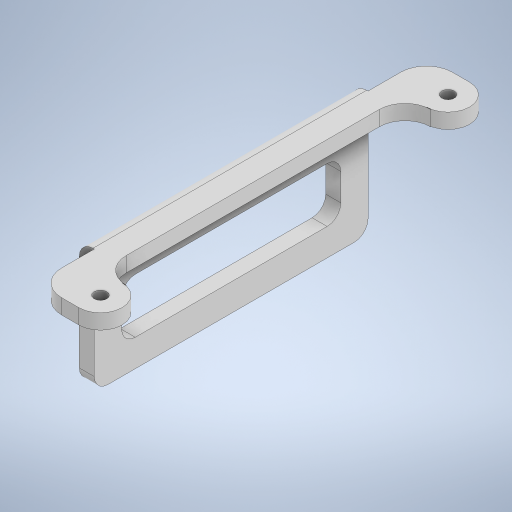
# Autodesk Inventor part: sidemount3
Saved by Autodesk Inventor 2023 (Build 270158000, 158)
## iProperties
Created: 2022-12-04
Part Number: sidemount3
Material: Generic
Document SubType Name: Modeling
Designer: user
Density: 1 g/cm^3
Appearance: Default
Author: user
Autodesk Inventor part; units mm, degrees
ref_plane "YZ Plane" through (0, 0, 0) normal (1, 0, 0) x (0, 1, 0)
ref_plane "XZ Plane" through (0, 0, 0) normal (0, 1, 0) x (-1, 0, 0)
ref_plane "XY Plane" through (0, 0, 0) normal (0, 0, 1) x (1, 0, 0)
sketch "Sketch1" plane through (0, 0, 0) normal (0, 1, 0) x (-1, 0, 0)
  circle A0 centre (0, 0) radius 1.4732
  circle A1 centre (0, -80.9498) radius 1.4732
  circle A2 centre (0, 0) radius 5.0165
  circle A3 centre (0, -80.9498) radius 5.0165
  line L0 (0, 5.0165) -> (4.033, 5.0165)
  line L1 (4.033, -85.9663) -> (0, -85.9663)
  line L2 (10.033, -79.9663) -> (10.033, -0.9835)
  line L3 (0, -5.0165) -> (-0.9835, -5.0165)
  line L4 (5.0165, -11.0165) -> (5.0165, -69.9333)
  line L5 (-0.9835, -75.9333) -> (0, -75.9333)
  arc A4 (10.033, -0.9835) -> (4.033, 5.0165) centre (4.033, -0.9835) ccw
  arc A5 (4.033, -85.9663) -> (10.033, -79.9663) centre (4.033, -79.9663) ccw
  arc A6 (5.0165, -11.0165) -> (-0.9835, -5.0165) centre (-0.9835, -11.0165) ccw
  arc A7 (-0.9835, -75.9333) -> (5.0165, -69.9333) centre (-0.9835, -69.9333) ccw
  point P0 (10.033, 5.0165)
  dimension "d0" = 2.9464
  dimension "d2" = 2.9464
  dimension "d3" = 10.033
  dimension "d4" = 10.033
  dimension "d7" = 80.9498
  dimension "d8" = 10.033
  dimension "d9" = 6
  dimension "d10" = 6
  dimension "d11" = 6
  dimension "d12" = 6
  constraints: 12 end point, 12 point on circle, 11 tangent, 8 centre point, 3 coincident, 2 perpendicular, 2 point on line, 1 horizontal
  measures "d0" diameter of A0
  measures "d2" diameter of A1
  measures "d3" diameter of A2
  measures "d4" diameter of A3
  measures "d7" distance of A2.centre A3.centre
  measures "d8" distance of L0.start point (10.033, 5.017)
  measures "d9" radius of A4
  measures "d10" radius of A5
  measures "d11" radius of A6
  measures "d12" radius of A7
extrude "Extrusion1" add sketch "Sketch1" along normal blind 3.5
sketch "Sketch2" plane through (-10.033, 0, -79.9663) normal (-1, 0, 0) x (0, 0, 1)
  line L0 (0, 0) -> (0, 3.5) projected
  line L1 (0, 0) -> (7.62, 0)
  line L2 (0, 0) -> (78.9828, 0) projected
  line L3 (7.62, 0) -> (7.62, -22.225)
  line L4 (7.62, 0) -> (71.374, 0)
  line L5 (68.9498, 0) -> (10.033, 0) projected
  line L6 (71.374, 0) -> (71.374, -22.225)
  line L7 (68.199, -25.4) -> (10.795, -25.4)
  line L8 (7.62, 0) -> (19.2419, 0) construction
  line L9 (71.374, 0) -> (44.6419, 0) construction
  line L10 (61.849, -6.35) -> (17.145, -6.35)
  line L11 (17.145, -19.05) -> (61.849, -19.05)
  line L12 (65.024, -15.875) -> (65.024, -9.525)
  line L13 (13.97, -9.525) -> (13.97, -15.875)
  arc A0 (17.145, -6.35) -> (13.97, -9.525) centre (17.145, -9.525) ccw
  arc A1 (65.024, -9.525) -> (61.849, -6.35) centre (61.849, -9.525) ccw
  arc A2 (61.849, -19.05) -> (65.024, -15.875) centre (61.849, -15.875) ccw
  arc A3 (13.97, -15.875) -> (17.145, -19.05) centre (17.145, -15.875) ccw
  arc A4 (7.62, -22.225) -> (10.795, -25.4) centre (10.795, -22.225) ccw
  arc A5 (68.199, -25.4) -> (71.374, -22.225) centre (68.199, -22.225) ccw
  point P0 (79.9663, 0)
  point P1 (7.62, -25.4)
  point P2 (13.97, -6.35)
  point P3 (71.374, 0)
  dimension "d15" = 7.62
  dimension "d16" = 25.4
  dimension "d17" = 63.754
  dimension "d19" = 6.35
  dimension "d22" = 3.175
  dimension "d23" = 3.175
  dimension "d24" = 3.175
  dimension "d25" = 3.175
  dimension "d26" = 3.175
  dimension "d27" = 3.175
  dimension "d33" = 44.704
  dimension "d34" = 44.704
  constraints: 22 end point, 12 point on circle, 12 tangent, 6 centre point, 6 point on line, 4 horizontal, 2 perpendicular, 2 vertical, 1 parallel
  measures "d15" distance of L0.start L1.end
  measures "d16" distance of L1.end point (7.62, -25.4)
  measures "d17" distance of L1.end L4.end
  measures "d19" horizontal distance of L1.end point (13.97, -6.35)
  measures "d22" radius of A0
  measures "d23" radius of A1
  measures "d24" radius of A2
  measures "d25" radius of A3
  measures "d26" radius of A4
  measures "d27" radius of A5
  measures "d33" distance of L10.start L10.end
  measures "d34" distance of L11.start L11.end
extrude "Extrusion2" add sketch "Sketch2" along normal blind 3.5
sketch "Sketch4" plane through (-10.033, 0, -8.5923) normal (0, 1, 0) x (1, 0, 0)
  line L0 (0, 63.754) -> (-3.5, 63.754) projected
  line L1 (0, 63.754) -> (-3.5, 63.754)
  line L2 (0, 0) -> (-3.5, 0) projected
  line L3 (-3.5, 63.754) -> (-3.5, 0)
  line L4 (-3.5, 0) -> (0, 0)
  line L5 (0, 0) -> (0, 63.754)
  point P0 (10.033, -8.5923)
  constraints: 8 end point, 2 perpendicular, 1 collinear, 1 horizontal
extrude "Extrusion3" add sketch "Sketch4" along normal blind 3.5
fillet "Fillet1" radius 3.175 1 edges at (-13.533, 3.5, -40.4693)
body "Solid1"
